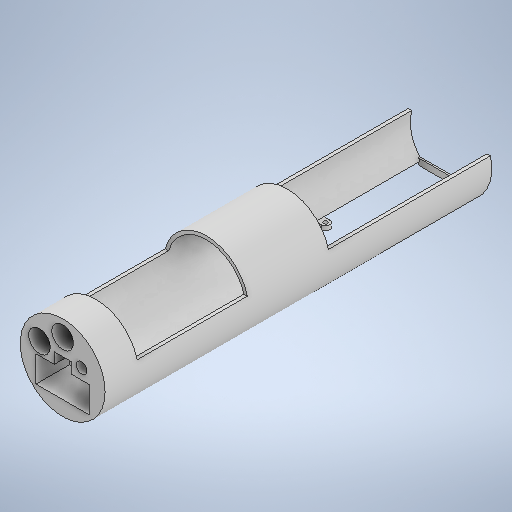
# Autodesk Inventor part: PCB tray CAD
Saved by Autodesk Inventor 2025 (Build 290162000, 162)
## iProperties
Created: 2024-07-01
Part Number: PCB tray CAD
Material: Generic
Document SubType Name: Modeling
Designer: track
Density: 1 g/cm^3
Appearance: Default
Author: track
## iProperties of the stored document PCB tray CAD_3DPrint.ipt
Created: 2024-07-01
Part Number: PCB tray CAD_3DPrint
Material: Generic
Document SubType Name: Modeling
Designer: track
Density: 1 g/cm^3
Appearance: Default
Author: track
Autodesk Inventor part; units mm, degrees
ref_plane "YZ Plane" through (0, 0, 0) normal (1, 0, 0) x (0, 1, 0)
ref_plane "XY Plane" through (0, 0, 0) normal (0, 0, 1) x (1, 0, 0)
sketch "Sketch9" plane through (0, 0, 0) normal (0, 0, 1) x (1, 0, 0)
  circle A0 centre (0, 0) radius 25.4
  circle A1 centre (0, 0) radius 23.4
  dimension "d29" = 50.8
  dimension "d30" = 2
  constraints: 2 centre point, 2 coincident
  measures "d29" diameter of A0
  measures "d30" radial gap between concentric circles of A0 A1
extrude "Extrusion7" add sketch "Sketch9" against normal blind 231.5
sketch "Sketch10" plane through (0, 0, 0) normal (0, 0, 1) x (1, 0, 0)
  circle A0 centre (0, 15.875) radius 6.5
  circle A1 centre (-13.89, 6.835) radius 6.5
  circle A2 centre (11.35, 5.565) radius 3.25
  line L0 (-16, -16.535) -> (-16, -0.785)
  line L1 (-16, -0.785) -> (-5, -0.785)
  line L2 (-5, -0.785) -> (-5, 5.715)
  line L3 (-5, 5.715) -> (5, 5.715)
  line L4 (5, 5.715) -> (5, -0.785)
  line L5 (5, -0.785) -> (16, -0.785)
  line L6 (16, -0.785) -> (16, -16.535)
  line L7 (16, -16.535) -> (-16, -16.535)
  line L8 (0, 5.715) -> (0, -16.535) construction
  circle A3 centre (0, 0) radius 23.4 projected
  dimension "d33" = 13
  dimension "d34" = 13
  dimension "d35" = 6.5
  dimension "d36" = 32
  dimension "d37" = 10
  dimension "d39" = 16
  dimension "d40" = 15.75
  dimension "d41" = 6.5
  dimension "d43" = 5.715
  dimension "d44" = 0
  dimension "d45" = 8.89
  dimension "d46" = 7.62
  dimension "d47" = 0
  dimension "d48" = 10.16
  dimension "d49" = 6.35
  dimension "d50" = 6.35
  constraints: 18 end point, 6 perpendicular, 3 centre point, 2 midpoint, 2 point on line, 2 vertical
  measures "d33" diameter of A0
  measures "d34" diameter of A1
  measures "d35" diameter of A2
  measures "d36" distance between parallel lines of L6 L0
  measures "d37" distance of L2.end L3.end
  measures "d39" distance between parallel lines of L6 L8
  measures "d40" distance of L5.end L6.end
  measures "d41" distance of L3.end L4.end
  measures "d43" distance of point (0, 0) L8.start
  measures "d44" distance from line of point (0, 0) L8
  measures "d45" distance from line of L2 A1.centre
  measures "d46" distance from line of L1 A1.centre
  measures "d47" distance from line of L8 A0.centre
  measures "d48" distance from line of L3 A0.centre
  measures "d49" distance from line of L5 A2.centre
  measures "d50" distance from line of L4 A2.centre
extrude "Extrusion8" add sketch "Sketch10" against normal blind 20
ref_plane "Work Plane1" through (0, 25.4, 0) normal (0, 1, 0) x (-1, 0, 0)
sketch "Sketch11" plane through (0, 25.4, 0) normal (0, 1, 0) x (-1, 0, 0)
  line L0 (-25.4, -231.5) -> (25.4, -231.5) projected
  line L1 (-25.4, 0) -> (-25.4, -231.5) projected
  line L2 (25.4, -231.5) -> (-25.4, -231.5)
  line L3 (-25.4, -231.5) -> (-25.4, -134.5)
  line L4 (-25.4, -134.5) -> (25.4, -134.5)
  line L5 (25.4, -134.5) -> (25.4, -231.5)
  point P0 (0, 0)
  dimension "d53" = 97
  constraints: 8 end point, 2 parallel, 1 horizontal, 1 perpendicular, 1 point on line
  measures "d53" distance of L4.end L0.end
extrude "Extrusion9" cut sketch "Sketch11" against normal blind 19.05
sketch "Sketch12" plane through (0, 0, -231.5) normal (0, 0, -1) x (-1, 0, 0)
  circle A0 centre (0, 0) radius 25.4 projected
  line L0 (-19.2809, -16.535) -> (19.2809, -16.535)
  line L1 (16, -16.535) -> (-16, -16.535) projected
  arc A1 (-19.2809, -16.535) -> (19.2809, -16.535) centre (0, 0) ccw
  dimension "d56" = 0
  constraints: 4 point on circle, 2 end point, 1 centre point, 1 concentric, 1 horizontal
  measures "d56" distance between parallel lines of L0 L1
extrude "Extrusion10" cut sketch "Sketch12" against normal blind 97 contours L0 A0 picked at (1.0399, -19.4259)
ref_plane "Work Plane3" through (0, -16.51, 0) normal (0, 1, 0) x (-1, 0, 0)
sketch "Sketch13" plane through (0, -16.51, 0) normal (0, 1, 0) x (-1, 0, 0)
  line L0 (0, 0) -> (0, -257.1233) construction
  line L1 (-16.5576, -231.5) -> (-16.5576, -134.5) projected
  line L2 (-16.5576, -134.5) -> (-13.0576, -134.5)
  line L3 (-13.0576, -134.5) -> (-13.0576, -139.5) construction
  line L4 (-13.0576, -139.5) -> (-16.5576, -139.5)
  line L5 (-16.5576, -139.5) -> (-16.5576, -134.5)
  line L6 (16.5576, -134.5) -> (16.5576, -231.5) projected
  line L7 (16.5576, -134.5) -> (13.0576, -134.5)
  line L8 (13.0576, -134.5) -> (13.0576, -139.5) construction
  line L9 (13.0576, -139.5) -> (16.5576, -139.5)
  line L10 (16.5576, -139.5) -> (16.5576, -134.5)
  line L11 (-16.5576, -168) -> (-13.0576, -168)
  line L12 (-13.0576, -168) -> (-13.0576, -173) construction
  line L13 (-13.0576, -173) -> (-16.5576, -173)
  line L14 (-16.5576, -173) -> (-16.5576, -168)
  line L15 (16.5576, -168) -> (13.0576, -168)
  line L16 (13.0576, -168) -> (13.0576, -173) construction
  line L17 (13.0576, -173) -> (16.5576, -173)
  line L18 (16.5576, -173) -> (16.5576, -168)
  arc A0 (-13.0576, -139.5) -> (-13.0576, -134.5) centre (-13.0576, -137) ccw
  arc A1 (13.0576, -134.5) -> (13.0576, -139.5) centre (13.0576, -137) ccw
  arc A2 (-13.0576, -173) -> (-13.0576, -168) centre (-13.0576, -170.5) ccw
  arc A3 (13.0576, -168) -> (13.0576, -173) centre (13.0576, -170.5) ccw
  circle A4 centre (-13.0576, -137) radius 1.25
  circle A5 centre (13.0576, -137) radius 1.25
  circle A6 centre (-13.0576, -170.5) radius 1.25
  circle A7 centre (13.0576, -170.5) radius 1.25
  point P0 (-10.5576, -137)
  point P1 (16.5576, -173)
  point P2 (16.5576, -168)
  dimension "d60" = 5
  dimension "d61" = 5
  dimension "d62" = 28.5
  dimension "d63" = 6
  dimension "d64" = 2.5
  dimension "d65" = 2.5
  constraints: 34 end point, 9 point on circle, 8 centre point, 8 parallel, 8 tangent, 5 point on line, 4 coincident, 4 horizontal, 4 perpendicular, 1 vertical, 6 other
  measures "d60" distance of L2.end L3.end
  measures "d61" distance of L11.end L12.end
  measures "d62" distance between parallel lines of L4 L11
  measures "d63" distance from line of L1 point (-10.558, -137)
  measures "d64" diameter of A4
  measures "d65" diameter of A6
extrude "Extrusion11" add sketch "Sketch13" against normal blind 2.54
sketch "Sketch14" plane through (0, 0, -134.5) normal (0, 0, -1) x (-1, 0, 0)
  line L0 (16.5576, -19.05) -> (13.5889, -19.05) projected
  arc A0 (-13.5889, -19.05) -> (13.5889, -19.05) centre (0, 0) ccw projected
  line L1 (-13.5889, -19.05) -> (-16.5576, -19.05) projected
  line L2 (-16.5576, -19.05) -> (-16.5576, -16.535) projected
  line L3 (-19.2809, -16.535) -> (-16.5576, -16.535) projected
  arc A1 (-19.2809, -16.535) -> (19.2809, -16.535) centre (0, 0) ccw projected
  line L4 (16.5576, -16.535) -> (19.2809, -16.535) projected
  line L5 (16.5576, -16.535) -> (16.5576, -19.05) projected
  line L6 (13.0576, -16.51) -> (13.0576, -19.05) projected
  line L7 (13.0576, -19.05) -> (16.8005, -19.05)
  line L8 (-13.0576, -16.51) -> (-13.0576, -19.05) projected
  line L9 (-13.0576, -19.05) -> (-16.8005, -19.05)
  point P0 (-16.5576, -19.2615)
  point P1 (16.5576, -19.2615)
  constraints: 4 end point, 4 point on circle, 3 point on line, 1 perpendicular
extrude "Extrusion12" add sketch "Sketch14" along normal up to surface (38.5 mm away) contours L5 L4 A1 L7 | A1 L3 L2 L9
sketch "Sketch15" plane through (0, 25.4, 0) normal (0, 1, 0) x (-1, 0, 0)
  line L0 (-25.4, 0) -> (-25.4, -231.5) projected
  line L1 (25.4, 0) -> (25.4, -231.5) projected
  line L2 (-25.4, -20) -> (25.4, -20)
  line L3 (25.4, -20) -> (25.4, -86)
  line L4 (25.4, -86) -> (-25.4, -86)
  line L5 (-25.4, -86) -> (-25.4, -20)
  line L6 (23.4, -20) -> (-23.4, -20) projected
  point P0 (0, 0)
  point P1 (-25.4, -86)
  point P2 (25.4, -20)
  dimension "d70" = 0
  dimension "d71" = 66
  constraints: 8 end point, 2 parallel, 2 point on line, 1 horizontal, 1 perpendicular
  measures "d70" distance between parallel lines of L6 L2
  measures "d71" distance between parallel lines of L2 L4
extrude "Extrusion13" cut sketch "Sketch15" against normal up to surface (19.05 mm away)
sketch "Sketch17" plane through (0, 0, -231.5) normal (0, 0, -1) x (-1, 0, 0)
  circle A0 centre (0, 0) radius 25.4
  arc A1 (-16.8005, -19.05) -> (16.8005, -19.05) centre (0, 0) ccw projected
  line L0 (-19.2809, -16.535) -> (-16.5576, -16.535) projected
  line L1 (-20.32, -15.24) -> (20.32, -15.24)
  line L2 (16.5576, -19.05) -> (13.0576, -19.05) projected
  line L3 (-16.8005, -19.05) -> (16.8005, -19.05)
  point P0 (16.8005, -19.05)
  dimension "d74" = 3.81
  constraints: 4 end point, 2 parallel, 2 point on circle, 1 centre point, 1 coincident, 1 concentric
  measures "d74" distance between parallel lines of L1 L3
extrude "Extrusion14" add sketch "Sketch17" against normal blind 1 contours L1 A0 L3 L2
body "Solid2"
